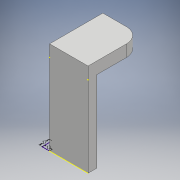
# Autodesk Inventor part: YETTOCOMPLETE
Saved by Autodesk Inventor 2017 (Build 210142000, 142)
## iProperties
Created: 2019-09-19
Part Number: YETTOCOMPLETE
Material: Generic
Document SubType Name: Modeling
Designer: Manan
Density: 1 g/cm^3
Appearance: Default
Author: Manan
Autodesk Inventor part; units mm, degrees
ref_plane "YZ Plane" through (0, 0, 0) normal (1, 0, 0) x (0, 1, 0)
ref_plane "XZ Plane" through (0, 0, 0) normal (0, 1, 0) x (-1, 0, 0)
ref_plane "XY Plane" through (0, 0, 0) normal (0, 0, 1) x (1, 0, 0)
sketch "Sketch1" plane through (0, 0, 0) normal (0, 0, 1) x (1, 0, 0)
  line L0 (0, 0) -> (65, 0)
  line L1 (65, 0) -> (65, 90)
  line L2 (65, 90) -> (0, 90)
  line L3 (0, 90) -> (0, 0)
  dimension "d0" = 65
  dimension "d1" = 90
  constraints: 8 end point, 2 parallel, 1 horizontal, 1 perpendicular
  measures "d0" distance of L2.end L1.end
  measures "d1" distance of L1.end L0.end
extrude "Extrusion1" add sketch "Sketch1" along normal blind 20
fillet "Fillet1" radius 25 1 edges at (65, 90, 10)
sketch "Sketch2" plane through (0, 0, 0) normal (0, 0, -1) x (-1, 0, 0)
  point P0 (0, 0)
sketch "Sketch3" plane through (65, 0, 20) normal (1, 0, 0) x (0, 0, -1)
  point P0 (20, 0)
sketch "Sketch4" plane through (0, 0, 0) normal (0, 0, -1) x (-1, 0, 0)
  point P0 (0, 0)
sketch "Sketch5" plane through (0, 0, 0) normal (0, -1, 0) x (1, 0, 0)
  line L0 (40, 0) -> (0, 0) projected
  line L1 (0, 0) -> (65, 0)
  line L2 (65, 0) -> (65, -137)
  line L3 (65, -137) -> (0, -137)
  line L4 (0, -137) -> (0, 0)
  dimension "d5" = 65
  dimension "d6" = 137
  constraints: 8 end point, 2 parallel, 1 horizontal, 1 perpendicular
  measures "d5" distance of L2.end L3.end
  measures "d6" distance of L1.end L2.end
extrude "Extrusion2" add sketch "Sketch5" against normal blind 15
sketch "Sketch6" plane through (65, 0, -137) normal (0, 0, -1) x (-1, 0, 0)
  line L0 (65, 0) -> (0, 0) projected
  line L1 (65, 0) -> (78, 0)
  line L2 (78, 0) -> (78, 17)
  line L3 (78, 17) -> (65, 0)
  dimension "d9" = 13
  dimension "d10" = 17
  constraints: 6 end point, 1 horizontal, 1 perpendicular
  measures "d9" distance of L0.start L1.end
  measures "d10" distance of L1.end L2.end
sketch "Sketch7" plane through (65, 0, -137) normal (0, 0, -1) x (-1, 0, 0)
  point P0 (65, 0)
body "Solid1"
